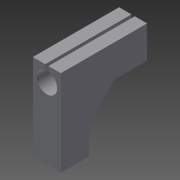
# Autodesk Inventor part: ZCarriageV1
Saved by Autodesk Inventor 2015 (Build 190159000, 159)
## iProperties
Created: 2014-08-22
Part Number: ZCarriageV1
Material: Generic
Document SubType Name: Modeling
Designer: t_clevj
Density: 1 g/cm^3
Appearance: Default
Author: t_clevj
Autodesk Inventor part; units mm, degrees
ref_plane "YZ Plane" through (0, 0, 0) normal (1, 0, 0) x (0, 1, 0)
ref_plane "XZ Plane" through (0, 0, 0) normal (0, 1, 0) x (-1, 0, 0)
ref_plane "XY Plane" through (0, 0, 0) normal (0, 0, 1) x (1, 0, 0)
sketch "Sketch1" plane through (0, 0, 0) normal (0, 1, 0) x (-1, 0, 0)
  arc A0 (-1.5, 9.3808) -> (1.5, 9.3808) centre (0, 0) ccw
  line L0 (1.5, 9.3808) -> (1.5, 14)
  line L1 (1.5, 14) -> (13, 14)
  line L2 (13, 14) -> (13, -16)
  line L3 (13, -16) -> (-13, -16)
  line L4 (-13, -16) -> (-13, 14)
  line L5 (-13, 14) -> (-1.5, 14)
  line L6 (-1.5, 14) -> (-1.5, 9.3808)
  dimension "d0" = 19
  dimension "d1" = 1.5
  dimension "d2" = 1.5
  dimension "d3" = 13
  dimension "d4" = 13
  dimension "d5" = 16
  dimension "d6" = 14
  constraints: 14 end point, 5 perpendicular, 2 point on circle, 2 point on line, 1 centre point, 1 coincident, 1 vertical
  measures "d0" diameter of A0
  measures "d1" distance from line of point (0, 0) L6
  measures "d2" distance from line of point (0, 0) L0
  measures "d3" distance from line of point (0, 0) L4
  measures "d4" distance from line of L2 point (0, 0)
  measures "d5" distance from line of point (0, 0) L3
  measures "d6" distance from line of L1 point (0, 0)
extrude "Extrusion1" add sketch "Sketch1" along normal blind 80
sketch "Sketch3" plane through (13, 0, 14) normal (1, 0, 0) x (0, 0, -1)
  line L0 (30, 0) -> (30, 80) projected
  line L1 (30, 0) -> (30, 80) projected
  line L2 (30, 50) -> (54, 26)
  line L3 (54, 26) -> (80, 26)
  line L4 (80, 26) -> (80, 0)
  line L5 (80, 0) -> (30, 0)
  point P0 (14, 0)
  dimension "d10" = 45
  dimension "d11" = 26
  dimension "d12" = 50
  dimension "d13" = 26
  constraints: 8 end point, 3 perpendicular, 1 point on line
  measures "d10" angle of L0 L2
  measures "d11" distance between parallel lines of L5 L3
  measures "d12" distance between parallel lines of L0 L4
  measures "d13" distance of L2.end L3.end
extrude "Extrusion2" add sketch "Sketch3" against normal up to surface (26 mm away)
sketch "Sketch4" plane through (13, 0, -66) normal (0, 0, -1) x (-1, 0, 0)
  line L0 (0, 0) -> (0, 26) projected
  line L1 (0, 0) -> (26, 0) projected
  line L2 (3, 3) -> (23, 3)
  line L3 (23, 3) -> (23, 23)
  line L4 (23, 23) -> (3, 23)
  line L5 (3, 23) -> (3, 3)
  point P0 (13, 0)
  dimension "d16" = 20
  dimension "d17" = 20
  dimension "d18" = 3
  dimension "d19" = 3
  constraints: 8 end point, 2 parallel, 1 horizontal, 1 perpendicular
  measures "d16" distance of L4.end L3.end
  measures "d17" distance of L3.end L2.end
  measures "d18" distance between parallel lines of L0 L5
  measures "d19" distance between parallel lines of L1 L2
extrude "Extrusion3" cut sketch "Sketch4" against normal blind 45
body "Solid1"
